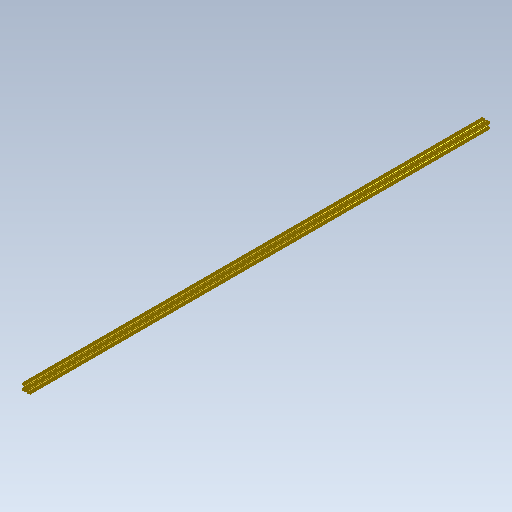
# Autodesk Inventor part: Perfil 30×30 4 rasgos ligeiro_AST03003004L
Saved by Autodesk Inventor 2025.2 (Build 292293000, 293)
## iProperties
Created: 2025-04-06
Part Number: Perfil 30×30 4 rasgos ligeiro_AST03003004L
Material: Ouro
Document SubType Name: Modeling
Designer: Gustavo Sousa
Density: 19.3 g/cm^3
Appearance: Metal quente 2400F
Author: Gustavo Sousa
Autodesk Inventor part; units mm, degrees
ref_plane "YZ Plane" through (0, 0, 0) normal (1, 0, 0) x (0, 1, 0)
ref_plane "XZ Plane" through (0, 0, 0) normal (0, 1, 0) x (-1, 0, 0)
ref_plane "XY Plane" through (0, 0, 0) normal (0, 0, 1) x (1, 0, 0)
sketch "Esboço1" plane through (0, 0, 0) normal (0, 0, 1) x (1, 0, 0)
  circle A0 centre (0, 0) radius 5 construction
  circle A1 centre (0, 0) radius 7.2 construction
  line L0 (-15, 15) -> (15, 15) construction
  line L1 (-15, 15) -> (0, 0) construction
  circle A2 centre (0, 0) radius 4.5 construction
  line L2 (-1.1, 4.5) -> (1.1, 4.5)
  line L3 (-1.1, 4.8775) -> (-1.1, 4.5)
  line L4 (1.1, 4.5) -> (1.1, 4.8775)
  line L5 (-4.2267, 2.6711) -> (-3.9598, 2.4042)
  line L6 (-3.9598, 2.4042) -> (-2.4042, 3.9598)
  line L7 (-2.4042, 3.9598) -> (-2.6711, 4.2267)
  line L8 (-4.8775, -1.1) -> (-4.5, -1.1)
  line L9 (-4.5, -1.1) -> (-4.5, 1.1)
  line L10 (-4.5, 1.1) -> (-4.8775, 1.1)
  line L11 (-2.6711, -4.2267) -> (-2.4042, -3.9598)
  line L12 (-2.4042, -3.9598) -> (-3.9598, -2.4042)
  line L13 (-3.9598, -2.4042) -> (-4.2267, -2.6711)
  line L14 (1.1, -4.8775) -> (1.1, -4.5)
  line L15 (1.1, -4.5) -> (-1.1, -4.5)
  line L16 (-1.1, -4.5) -> (-1.1, -4.8775)
  line L17 (4.2267, -2.6711) -> (3.9598, -2.4042)
  line L18 (3.9598, -2.4042) -> (2.4042, -3.9598)
  line L19 (2.4042, -3.9598) -> (2.6711, -4.2267)
  line L20 (4.8775, 1.1) -> (4.5, 1.1)
  line L21 (4.5, 1.1) -> (4.5, -1.1)
  line L22 (4.5, -1.1) -> (4.8775, -1.1)
  line L23 (2.6711, 4.2267) -> (2.4042, 3.9598)
  line L24 (2.4042, 3.9598) -> (3.9598, 2.4042)
  line L25 (3.9598, 2.4042) -> (4.2267, 2.6711)
  arc A3 (-1.1, 4.8775) -> (-2.6711, 4.2267) centre (0, 0) ccw
  arc A4 (-4.2267, 2.6711) -> (-4.8775, 1.1) centre (0, 0) ccw
  arc A5 (-4.8775, -1.1) -> (-4.2267, -2.6711) centre (0, 0) ccw
  arc A6 (-2.6711, -4.2267) -> (-1.1, -4.8775) centre (0, 0) ccw
  arc A7 (1.1, -4.8775) -> (2.6711, -4.2267) centre (0, 0) ccw
  arc A8 (4.2267, -2.6711) -> (4.8775, -1.1) centre (0, 0) ccw
  arc A9 (4.8775, 1.1) -> (4.2267, 2.6711) centre (0, 0) ccw
  arc A10 (2.6711, 4.2267) -> (1.1, 4.8775) centre (0, 0) ccw
  line L26 (0, 6.5) -> (-1.1, 7.1155)
  line L27 (0, 6.5) -> (1.1, 7.1155)
  line L28 (-6.5, 0) -> (-7.1155, -1.1)
  line L29 (-6.5, 0) -> (-7.1155, 1.1)
  line L30 (0, -6.5) -> (1.1, -7.1155)
  line L31 (0, -6.5) -> (-1.1, -7.1155)
  line L32 (6.5, 0) -> (7.1155, 1.1)
  line L33 (6.5, 0) -> (7.1155, -1.1)
  line L34 (-4.1, 15) -> (4.1, 15)
  line L35 (-4.1, 15) -> (-4.6, 15) construction
  line L36 (-4.6, 15) -> (-4.6, 14.5)
  line L37 (-4.6, 14.5) -> (-4.1, 14.5)
  line L38 (-4.1, 14.5) -> (-4.1, 15) construction
  line L39 (-4.6, 15) -> (-5.1942, 15)
  line L40 (-15, 15) -> (-15, -15) construction
  arc A11 (-14.5, 15) -> (-15, 14.5) centre (-14.5, 14.5) ccw construction
  line L41 (-14.5, 15) -> (-5.1942, 15)
  arc A12 (-14.5, 15) -> (-14.8536, 14.8536) centre (-14.5, 14.5) ccw
  line L42 (-4.1, 15) -> (-4.1, 12.8) construction
  line L43 (-4.1, 12.8) -> (-8.15, 12.8) construction
  line L44 (-4.1, 14.5) -> (-4.1, 12.8)
  line L45 (-8.15, 12.8) -> (-8.15, 9.7056) construction
  line L46 (-13.75, 13.75) -> (-9.25, 13.75) construction
  line L47 (-9.25, 13.75) -> (-9.25, 9.25) construction
  line L48 (-9.25, 9.25) -> (-13.75, 9.25) construction
  line L49 (-13.75, 9.25) -> (-13.75, 13.75) construction
  line L50 (-13.75, 13.75) -> (-9.25, 9.25) construction
  line L51 (-9.25, 13.75) -> (-13.75, 9.25) construction
  line L52 (-8.15, 9.7056) -> (-4.2536, 5.8092) construction
  arc A13 (-1.1, 7.1155) -> (-4.2536, 5.8092) centre (0, 0) ccw construction
  line L53 (-4.2536, 5.8092) -> (-2.6711, 4.2267) construction
  arc A14 (7.1155, 1.1) -> (1.1, 7.1155) centre (0, 0) ccw
  arc A15 (1.1, -7.1155) -> (7.1155, -1.1) centre (0, 0) ccw
  arc A16 (-7.1155, -1.1) -> (-1.1, -7.1155) centre (0, 0) ccw
  arc A17 (-5.0912, 5.0912) -> (-7.1155, 1.1) centre (0, 0) ccw
  line L54 (-5.0912, 5.0912) -> (-9.25, 9.25)
  line L55 (-9.25, 9.25) -> (-13.75, 13.75)
  line L56 (-13.75, 13.75) -> (-14.8536, 14.8536)
  arc A18 (-4.5481, 6.1037) -> (-3.9221, 6.0379) centre (-4.1945, 6.4573) ccw
  arc A19 (-8.15, 9.9127) -> (-8.0036, 9.5592) centre (-7.65, 9.9127) ccw
  arc A20 (-7.65, 12.8) -> (-8.15, 12.3) centre (-7.65, 12.3) ccw
  line L57 (-7.65, 12.8) -> (-4.1, 12.8)
  line L58 (-8.15, 12.3) -> (-8.15, 9.9127)
  line L59 (-8.0036, 9.5592) -> (-4.5481, 6.1037)
  arc A21 (-1.1, 7.1155) -> (-3.9221, 6.0379) centre (0, 0) ccw
  arc A22 (-13.25, 13.75) -> (-13.75, 13.25) centre (-13.25, 13.25) ccw construction
  arc A23 (-9.25, 13.25) -> (-9.75, 13.75) centre (-9.75, 13.25) ccw
  arc A24 (-9.75, 9.25) -> (-9.25, 9.75) centre (-9.75, 9.75) ccw construction
  arc A25 (-13.25, 13.75) -> (-13.6036, 13.6036) centre (-13.25, 13.25) ccw
  line L60 (-13.25, 13.75) -> (-9.75, 13.75)
  arc A26 (-9.3964, 9.3964) -> (-9.25, 9.75) centre (-9.75, 9.75) ccw
  line L61 (-9.25, 13.25) -> (-9.25, 9.75)
  point P0 (0, 15)
  point P1 (0, 4.5)
  point P2 (-3.182, 3.182)
  point P3 (-4.5, 0)
  point P4 (-3.182, -3.182)
  point P5 (0, -4.5)
  point P6 (3.182, -3.182)
  point P7 (4.5, 0)
  point P8 (3.182, 3.182)
  point P9 (0, 15)
  point P10 (-11.5, 11.5)
  dimension "d14" = 9
  dimension "d0" = 10
  dimension "d2" = 30
  dimension "d3" = 15
  dimension "d10" = 360
  dimension "d15" = 2.2
  dimension "d17" = 2
  dimension "d19" = 2.2
  dimension "d24" = 360
  dimension "d26" = 8.2
  dimension "quadrado" = 0.5
  dimension "arco" = 0.5
  dimension "espessura" = 2.2
  dimension "d32" = 4.5
  dimension "d33" = 1.1
  dimension "d34" = 11.5
  constraints: 124 end point, 60 point on circle, 26 centre point, 23 equal radius, 21 tangent, 18 point on line, 8 collinear, 7 vertical alignment, 6 coincident, 6 horizontal, 5 midpoint, 5 parallel, 4 equal length, 4 vertical, 2 perpendicular, 1 concentric, 88 other
  measures "d0" diameter of A0
  measures "d2" distance of L0.start L0.end
  measures "d3" distance of point (0, 0) point (0, 15)
  measures "d15" distance between parallel lines of L3 L4
  measures "d17" distance of point (0, 4.5) L26.start
  measures "d19" radial gap between concentric circles of A10 A1
  measures "d26" distance of L34.start L34.end
  measures "quadrado" distance of L35.end L36.end
  measures "arco" radius of A11
  measures "espessura" distance between parallel lines of L43 L0
  measures "d32" distance of L46.start L46.end
  measures "d33" distance between parallel lines of L45 L47
  measures "d34" horizontal distance of A10.centre point (-11.5, 11.5)
extrude "Extrusão1" add sketch "Esboço1" along normal mid plane 2000 contours L27 A14 L32 L33 A15 L30 L31 A16 L28 L29 A17 L54 L55 A26 L61 A23 L60 A25 L56 A12 L41 L39 L36 L37 L44 L57 A20 L58 A19 L59 A18 A21 L26
mirror "Espelhar1" about plane through (-14.8536, 14.8536, 0) normal (-0.7071, -0.7071, 0) of "Extrusão1"
mirror "Espelhar2" about plane through (0, 0, 0) normal (0, 1, 0) of "Extrusão1", "Espelhar1"
mirror "Espelhar3" about plane through (0, 0, 0) normal (1, 0, 0) of "Extrusão1", "Espelhar1", "Espelhar2"
